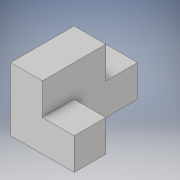
# Autodesk Inventor part: Substract Method(1)
Saved by Autodesk Inventor 2019 (Build 230136000, 136)
## iProperties
Created: 2019-09-05
Part Number: Substract Method(1)
Material: Generic
Document SubType Name: Modeling
Designer: IED8
Density: 1 g/cm^3
Appearance: Default
Author: IED8
Autodesk Inventor part; units mm, degrees
ref_plane "YZ Plane" through (0, 0, 0) normal (1, 0, 0) x (0, 1, 0)
ref_plane "XZ Plane" through (0, 0, 0) normal (0, 1, 0) x (-1, 0, 0)
ref_plane "XY Plane" through (0, 0, 0) normal (0, 0, 1) x (1, 0, 0)
sketch "Sketch1" plane through (0, 0, 0) normal (1, 0, 0) x (0, 1, 0)
  line L0 (0, -48.94) -> (-38.1, -48.94)
  line L1 (-38.1, -48.94) -> (-38.1, 8.21)
  line L2 (-38.1, 8.21) -> (0, 8.21)
  line L3 (0, 8.21) -> (0, -48.94)
  point P0 (0, 0)
  dimension "d1" = 38.1
  dimension "d2" = 57.15
  constraints: 8 end point, 1 perpendicular, 1 vertical
  measures "d1" distance of L0.start L0.end
  measures "d2" distance of L0.end L1.end
extrude "Extrusion1" add sketch "Sketch1" along normal blind 38.1
sketch "Sketch2" plane through (38.1, 0, 0) normal (1, 0, 0) x (0, 0, -1)
  line L0 (-8.21, 0) -> (-8.21, -38.1) projected
  line L1 (-8.21, 0) -> (-8.21, -19.05)
  line L2 (-8.21, -19.05) -> (10.84, -19.05)
  line L3 (10.84, -19.05) -> (10.84, -38.1)
  line L4 (-8.21, -38.1) -> (48.94, -38.1) projected
  line L5 (48.94, -38.1) -> (48.94, 0) projected
  line L6 (10.84, -38.1) -> (48.94, -38.1)
  line L7 (48.94, -38.1) -> (48.94, 0)
  line L8 (48.94, 0) -> (-8.21, 0) projected
  line L9 (48.94, 0) -> (-8.21, 0)
  point P0 (0, 0)
  dimension "d5" = 19.05
  dimension "d6" = 19.05
  constraints: 12 end point, 3 perpendicular, 1 collinear, 1 horizontal, 1 midpoint, 1 point on line
  measures "d5" distance of L0.start L1.end
  measures "d6" distance of L1.end L2.end
extrude "Extrusion2" cut sketch "Sketch2" against normal blind 19.05 contours L8 L5 L4 L3 L2 L0
sketch "Sketch3" plane through (19.05, 0, 0) normal (1, 0, 0) x (0, 0, -1)
  line L0 (48.94, 0) -> (48.94, -38.1) projected
  line L1 (48.94, 0) -> (29.89, 0)
  line L2 (-8.21, 0) -> (48.94, 0) projected
  line L3 (29.89, 0) -> (29.89, -19.05)
  line L4 (29.89, -19.05) -> (48.94, -19.05)
  line L5 (48.94, -19.05) -> (48.94, 0)
  point P0 (0, 0)
  dimension "d9" = 19.05
  dimension "d10" = 19.05
  constraints: 8 end point, 3 perpendicular, 1 point on line
  measures "d9" distance of L0.start L1.end
  measures "d10" distance of L1.end L3.end
extrude "Extrusion3" cut sketch "Sketch3" against normal blind 19.05
body "Solid1"
